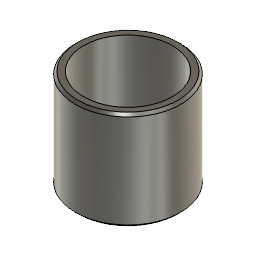
alkane-lamp-connector-pipe-43mm (Autodesk Fusion 360 design; units mm, degrees)
Autodesk Fusion 360 part; units mm, degrees
sketch "Skizze1" plane through (0, 0, 0) normal (0, 0, 1) x (1, 0, 0)
  circle A0 centre (0, 0) radius 18
  circle A1 centre (0, 0) radius 21.4
extrude "Extrusion1" add sketch "Skizze1" along normal blind 40
chamfer "Fase1" distance 1 angle 45 2 edges at (-19.9518, -7.7386, 40) (-19.9518, -7.7386, 0) tangent chain off
equation "outer_diameter = 42.80 mm" comment "Außendurchmesser des Rohres (43mm Nennmaß - 0.20mm Spiel)"
equation "inner_diameter = 36 mm" comment "Innendurchmesser des Rohres"
equation "pipe_length = 40 mm" comment "Gesamtlänge des Verbindungsrohres"
equation "outer_chamfer = 1 mm" comment "Fase an den äußeren Kanten des Rohres"
equation "d5 = pipe_length"
equation "d7 = outer_chamfer"
named bodies: "connector-pipe-43mm"
